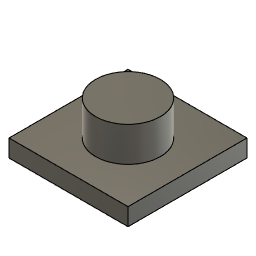
button (Autodesk Fusion 360 design; units mm, degrees)
Autodesk Fusion 360 part; units mm, degrees
sketch "Schizzo1" plane through (0, 0, 0) normal (0, 1, 0) x (1, 0, 0)
  line L0 (19.547, -15.8464) -> (25.847, -15.8464)
  line L1 (25.847, -15.8464) -> (25.847, -22.1464)
  line L2 (25.847, -22.1464) -> (19.547, -22.1464)
  line L3 (19.547, -22.1464) -> (19.547, -15.8464)
  line L4 (27.847, -24.1464) -> (17.547, -24.1464)
  line L5 (17.547, -24.1464) -> (17.547, -13.8464)
  line L6 (17.547, -13.8464) -> (27.847, -13.8464)
  line L7 (27.847, -13.8464) -> (27.847, -24.1464)
  dimension "d1" = 6.3
  dimension "d2" = 6.3
  dimension "d3" = -2
  constraint horizontal L0
  constraint vertical L1
  constraint horizontal L2
  constraint vertical L3
  measures "d1" distance of L0.start L0.end
  measures "d2" distance of L0.start L2.end
extrude "Estrusione1" add sketch "Schizzo1" along normal blind 2 contours L0 L1 L2 L3 | L4 L5 L6 L7
extrude "Estrusione2" add sketch "Schizzo1" along normal blind 7 contours L0 L1 L2 L3
extrude "Estrusione3" cut 1 faces at (21.647, 7, 17.9464) along direction (0, -1, 0) blind 2
move_face "FacceDiOffset1" offset -0.15 4 faces at (21.647, 3, 15.8464) (19.547, 3, 20.0464) (23.747, 3, 22.1464) (25.847, 3, 17.9464)
extrude "Estrusione4" cut 1 faces at (25.697, 4, 19.9964) along direction (-1, 0, 0) blind 0.2
extrude "Estrusione5" cut 1 faces at (23.5637, 3, 15.9964) along direction (0, 0, 1) blind 0.2
extrude "Estrusione6" cut 1 faces at (19.697, 3, 20.063) along direction (1, 0, 0) blind 0.2
extrude "Estrusione7" cut 1 faces at (23.6304, 4, 21.9964) along direction (0, 0, -1) blind 0.2
extrude "Estrusione8" cut 1 faces at (24.4137, 0, 17.2797) along direction (0, 1, 0) blind 0.5
sketch "Schizzo2" plane through (0, 5, 0) normal (0, 1, 0) x (-1, 0, 0)
  line L0 (-19.897, 21.7964) -> (-25.497, 21.7964)
  line L1 (-25.497, 21.7964) -> (-25.497, 16.1964)
  line L2 (-25.497, 16.1964) -> (-19.897, 16.1964)
  line L3 (-19.897, 16.1964) -> (-19.897, 21.7964)
  circle A0 centre (-22.697, 18.9964) radius 2.8
  constraint tangent L1 A0
extrude "Estrusione9" cut sketch "Schizzo2" against normal blind 3 contours L0 L3 A0 | L0 L1 A0 | L2 L3 A0 | L1 L2 A0
